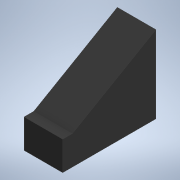
# Autodesk Inventor part: cabinet
Saved by Autodesk Inventor 2020 (Build 240168000, 168)
## iProperties
Created: 2021-03-06
Part Number: cabinet
Material: Generic
Document SubType Name: Modeling
Designer: Harry
Density: 1 g/cm^3
Appearance: Rubber - Black
Author: Harry
Autodesk Inventor part; units mm, degrees
ref_plane "YZ Plane" through (0, 0, 0) normal (1, 0, 0) x (0, 1, 0)
ref_plane "XZ Plane" through (0, 0, 0) normal (0, 1, 0) x (-1, 0, 0)
ref_plane "XY Plane" through (0, 0, 0) normal (0, 0, 1) x (1, 0, 0)
sketch "Sketch1" plane through (0, 0, 0) normal (1, 0, 0) x (0, 1, 0)
  line L0 (0, 0) -> (500, -866.0254)
  line L1 (0, 0) -> (1000, 0) construction
  line L2 (0, 0) -> (0, 100)
  line L3 (0, 100) -> (-300, 100)
  line L4 (-300, 100) -> (-300, -866.0254)
  line L5 (500, -866.0254) -> (-300, -866.0254)
  dimension "d0" = 1000
  dimension "d1" = 60
  dimension "d2" = 100
  dimension "d3" = 300
  constraints: 12 end point, 2 parallel, 1 equal length, 1 horizontal, 1 perpendicular, 1 vertical
  measures "d0" distance of L0.start L0.end
  measures "d1" angle of L0 L1
  measures "d2" distance of L0.start L2.end
  measures "d3" distance of L2.end L3.end
extrude "Extrusion1" add sketch "Sketch1" against normal blind 400
body "Solid1"
